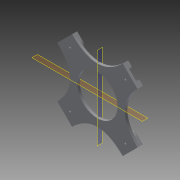
# Autodesk Inventor part: corps
Saved by Autodesk Inventor 2015 (Build 190159000, 159)
## iProperties
Created: 2015-02-17
Part Number: corps
Material: Generic
Document SubType Name: Modeling
Designer: Piotr
Density: 1 g/cm^3
Appearance: Default
Mass: 314.855 g
Surface Area: 705.583 cm^2
Volume: 314.855 cm^3
Author: Piotr
Autodesk Inventor part; units mm, degrees
ref_plane "YZ Plane" through (0, 0, 0) normal (1, 0, 0) x (0, 1, 0)
ref_plane "XZ Plane" through (0, 0, 0) normal (0, 1, 0) x (-1, 0, 0)
ref_plane "XY Plane" through (0, 0, 0) normal (0, 0, 1) x (1, 0, 0)
sketch "Sketch1" plane through (0, 0, 0) normal (0, 1, 0) x (-1, 0, 0)
  line L0 (80, 80) -> (-80, 80)
  line L1 (-80, 80) -> (-80, -80)
  line L2 (-80, -80) -> (80, -80)
  line L3 (80, -80) -> (80, 80)
  line L4 (0, 220.1005) -> (0, -177.8894) construction
  line L5 (-251.4311, 0) -> (-465.769, 0) construction
  point P0 (0, 0)
  dimension "d0" = 160
  dimension "d1" = 160
  constraints: 12 end point, 2 horizontal, 2 parallel, 2 point on line, 1 perpendicular, 1 vertical, 2 other
  measures "d0" distance of L2.end L0.start
  measures "d1" distance of L1.end L2.end
extrude "Extrusion1" add sketch "Sketch1" along normal blind 5
sketch "Sketch2" plane through (0, 5, 0) normal (0, 1, 0) x (1, 0, 0)
  line L0 (-80, -80) -> (80, -80) projected
  line L1 (80, -80) -> (80, 80) projected
  line L2 (80, 80) -> (-80, 80) projected
  line L3 (-80, 80) -> (-80, -80) projected
  line L4 (-80, -80) -> (80, -80) projected
  line L5 (-50.5, -80) -> (-80, -50.5)
  line L6 (-80, 80) -> (-80, -80) projected
  point P0 (0, 0)
  dimension "d4" = 45
  dimension "d5" = 29.5
  constraints: 2 end point, 2 point on line
  measures "d4" angle of L3 L5
  measures "d5" distance of L5.end L0.start
split body "Split1" sketch "Sketch2" result one side removed curves L5 removed pieces at (-70.1667, 0.5, 70.1667)
ref_plane "Work Plane1" through (80, 0, 0) normal (0, 0, 1) x (1, 0, 0)
ref_plane "Work Plane2" through (0, 0, -80) normal (-1, 0, 0) x (0, 0, 1)
mirror "Mirror1" about plane through (80, 0, 0) normal (0, 0, 1) of "Split1"
mirror "Mirror2" about plane through (0, 0, -80) normal (-1, 0, 0) of "Split1", "Mirror1"
sketch "Sketch4" plane through (0, 5, 0) normal (0, 1, 0) x (1, 0, 0)
  line L0 (80, 50.5) -> (50.5, 80) projected
  line L1 (65.25, 65.25) -> (45.1688, 45.1688) construction
  line L2 (80, 50.5) -> (70, 40.5)
  line L3 (70, 40.5) -> (38.811, 71.689) construction
  arc A0 (40.5, 70) -> (70, 40.5) centre (55.25, 55.25) ccw
  line L4 (50.5, 80) -> (40.5, 70)
  line L5 (40.5, 70) -> (71.689, 38.811) construction
  line L6 (50.5, 80) -> (80, 50.5)
  point P0 (0, 0)
  dimension "d6" = 10
  constraints: 12 end point, 2 perpendicular, 2 point on circle, 2 point on line, 1 centre point, 1 midpoint, 1 parallel, 1 symmetric about line
  measures "d6" horizontal distance of L0.start L2.end
extrude "Extrusion2" add sketch "Sketch4" along normal blind 6
sketch "Sketch5" plane through (0, 11, 0) normal (0, 1, 0) x (1, 0, 0)
  line L0 (80, 50.5) -> (50.5, 80) construction
  line L1 (50.5, 80) -> (40.5, 70) construction
  arc A0 (40.5, 70) -> (70, 40.5) centre (55.25, 55.25) ccw construction
  line L2 (70, 40.5) -> (80, 50.5) construction
  circle A1 centre (55.25, 55.25) radius 10 construction
  line L3 (62.3211, 48.1789) -> (72.3211, 58.1789)
  line L4 (48.1789, 62.3211) -> (58.1789, 72.3211)
  arc A2 (48.1789, 62.3211) -> (62.3211, 48.1789) centre (55.25, 55.25) ccw
  line L5 (72.3211, 58.1789) -> (58.1789, 72.3211)
  line L6 (80, 50.5) -> (50.5, 80) projected
  point P0 (0, 0)
  constraints: 6 end point, 4 point on circle, 2 centre point, 2 coincident, 2 collinear, 2 perpendicular, 1 tangent
extrude "Extrusion3" cut sketch "Sketch5" against normal blind 6
sketch "Sketch7" plane through (0, 5, 0) normal (0, 1, 0) x (1, 0, 0)
  circle A0 centre (55.25, 55.25) radius 5
  arc A1 (48.1789, 62.3211) -> (62.3211, 48.1789) centre (55.25, 55.25) ccw projected
  point P0 (0, 0)
  dimension "d11" = 10
  constraints: 1 centre point, 1 concentric
  measures "d11" diameter of A0
extrude "Extrusion4" cut sketch "Sketch7" against normal blind 3
hole "Hole1" at (55.25, 2, -55.25) direction (0, -1, 0) diameter 4 end through all
chamfer "Chamfer1" distance 1 angle 45 6 edges at (67.3211, 11, -53.1789) (48.1789, 11, -48.1789) (53.1789, 11, -67.3211) (75, 11, -45.5) (40.5, 11, -40.5) (45.5, 11, -75)
mirror "Mirror3" about plane through (0, 0, -80) normal (-1, 0, 0) of "Extrusion2", "Extrusion3", "Extrusion4", "Hole1", "Chamfer1"
mirror "Mirror4" about plane through (80, 0, 0) normal (0, 0, 1) of "Extrusion2", "Extrusion3", "Extrusion4", "Hole1", "Chamfer1", "Mirror3"
sketch "Sketch8" plane through (0, 5, 0) normal (0, 1, 0) x (1, 0, 0)
  line L0 (80, -50.5) -> (29.5, 0) construction
  line L1 (29.5, 0) -> (80, 50.5) construction
  spline S0 degree 2 poles (80, -50.5) (29.5, 0) (80, 50.5) knots 1 1 1 2 2 2
  line L2 (80, -50.5) -> (70, -40.5) projected
  line L3 (70, 40.5) -> (80, 50.5) projected
  line L4 (80, -50.5) -> (80, 50.5)
  line L5 (80, -50.5) -> (80, 50.5) projected
  point P0 (0, 0)
  constraints: 3 collinear, 2 end point, 3 other
extrude "Extrusion5" cut sketch "Sketch8" against normal blind 10
mirror "Mirror5" about plane through (0, 0, -80) normal (-1, 0, 0) of "Extrusion5"
sketch "Sketch9" plane through (0, 5, 0) normal (0, 1, 0) x (1, 0, 0)
  line L0 (-50.5, -80) -> (0, -29.5) construction
  line L1 (0, -29.5) -> (50.5, -80) construction
  spline S0 degree 2 poles (-50.5, -80) (0, -29.5) (50.5, -80) knots 1 1 1 2 2 2
  line L2 (-50.5, -80) -> (50.5, -80) projected
  line L3 (-50.5, -80) -> (-40.5, -70) projected
  line L4 (40.5, -70) -> (50.5, -80) projected
  point P0 (0, 0)
  constraints: 2 collinear, 3 other
extrude "Extrusion6" cut sketch "Sketch9" against normal blind 10
mirror "Mirror6" about plane through (80, 0, 0) normal (0, 0, 1) of "Extrusion6"
sketch "Sketch10" plane through (0, 5, 0) normal (0, 1, 0) x (1, 0, 0)
  circle A0 centre (0, 0) radius 40
  dimension "d30" = 80
  constraints: 1 centre point, 1 coincident
  measures "d30" diameter of A0
extrude "Extrusion7" cut sketch "Sketch10" against normal blind 10
body "Solid1"
